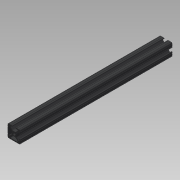
# Autodesk Inventor part: 1002
Saved by Autodesk Inventor 2013 (Build 170138000, 138)
## iProperties
Company: 80/20 Inc.
Created: 2013-09-06
Part Number: 1002
Material: Generic
Document SubType Name: Modeling
Density: 1 g/cm^3
Catalog Web Link: 8020.net
Vendor: 80/20 Inc.
Engineer: Ross Bowman
Author: Ross Bowman
Keywords: T-Slot, Extrusion, 80/20, 8020, Quick Frame, HT
Autodesk Inventor part; units mm, degrees
ref_plane "YZ Plane" through (0, 0, 0) normal (1, 0, 0) x (0, 1, 0)
ref_plane "XZ Plane" through (0, 0, 0) normal (0, 1, 0) x (-1, 0, 0)
ref_plane "XY Plane" through (0, 0, 0) normal (0, 0, 1) x (1, 0, 0)
sketch "Sketch1" plane through (0, 0, 0) normal (0, 0, 1) x (1, 0, 0)
  circle A0 centre (0, 0) radius 2.6035
  arc A1 (-8.737, 7.1292) -> (-10.4902, 6.4021) centre (-9.4628, 6.4021) ccw
  line L0 (-5.4405, 3.8388) -> (-8.737, 7.1292)
  arc A2 (-4.5085, 1.5917) -> (-5.4405, 3.8388) centre (-7.6835, 1.5917) ccw
  line L1 (-4.5085, -1.5917) -> (-4.5085, 1.5917)
  arc A3 (-5.4405, -3.8388) -> (-4.5085, -1.5917) centre (-7.6835, -1.5917) ccw
  line L2 (-8.7534, -7.1457) -> (-5.4405, -3.8388)
  arc A4 (-10.4902, -6.4254) -> (-8.7534, -7.1457) centre (-9.4724, -6.4254) ccw
  line L3 (-10.4902, 6.4021) -> (-10.4902, -6.4254)
  arc A5 (-7.1537, -8.6712) -> (-6.436, -10.4062) centre (-6.436, -9.3902) ccw
  line L4 (-3.9003, -5.4237) -> (-7.1537, -8.6712)
  arc A6 (-1.6573, -4.4958) -> (-3.9003, -5.4237) centre (-1.6573, -7.6708) ccw
  line L5 (1.6573, -4.4958) -> (-1.6573, -4.4958)
  arc A7 (3.9003, -5.4237) -> (1.6573, -4.4958) centre (1.6573, -7.6708) ccw
  line L6 (7.1478, -8.6653) -> (3.9003, -5.4237)
  arc A8 (6.4276, -10.4062) -> (7.1478, -8.6653) centre (6.4276, -9.3868) ccw
  line L7 (-6.436, -10.4062) -> (6.4276, -10.4062)
  arc A9 (6.3331, -12.7) -> (5.3171, -12.7) centre (5.8251, -12.7) ccw
  line L8 (6.3331, -12.7) -> (9.5504, -12.7)
  arc A10 (10.5664, -12.6998) -> (9.5504, -12.7) centre (10.0584, -12.7) ccw
  arc A11 (10.5664, -12.6998) -> (12.6998, -10.5664) centre (10.5918, -10.5918) ccw
  arc A12 (12.7, -9.5504) -> (12.6998, -10.5664) centre (12.7, -10.0584) ccw
  line L9 (12.7, -9.5504) -> (12.7, -6.3331)
  arc A13 (12.7, -5.3171) -> (12.7, -6.3331) centre (12.7, -5.8251) ccw
  line L10 (12.7, -5.3171) -> (12.7, -4.2875)
  arc A14 (12.7, -4.2875) -> (11.651, -3.2385) centre (11.651, -4.2875) ccw
  line L11 (11.651, -3.2385) -> (11.5392, -3.2385)
  arc A15 (11.5392, -3.2385) -> (10.4902, -4.2875) centre (11.5392, -4.2875) ccw
  line L12 (10.4902, -4.2875) -> (10.4902, -6.4021)
  arc A16 (8.737, -7.1292) -> (10.4902, -6.4021) centre (9.4628, -6.4021) ccw
  line L13 (8.737, -7.1292) -> (5.4405, -3.8388)
  arc A17 (4.5085, -1.5917) -> (5.4405, -3.8388) centre (7.6835, -1.5917) ccw
  line L14 (4.5085, -1.5917) -> (4.5085, 1.5917)
  arc A18 (5.4405, 3.8388) -> (4.5085, 1.5917) centre (7.6835, 1.5917) ccw
  line L15 (5.4405, 3.8388) -> (8.737, 7.1292)
  arc A19 (10.4902, 6.4021) -> (8.737, 7.1292) centre (9.4628, 6.4021) ccw
  line L16 (10.4902, 6.4021) -> (10.4902, 4.2875)
  arc A20 (10.4902, 4.2875) -> (11.5392, 3.2385) centre (11.5392, 4.2875) ccw
  line L17 (11.5392, 3.2385) -> (11.651, 3.2385)
  arc A21 (11.651, 3.2385) -> (12.7, 4.2875) centre (11.651, 4.2875) ccw
  line L18 (12.7, 4.2875) -> (12.7, 5.3171)
  arc A22 (12.7, 6.3331) -> (12.7, 5.3171) centre (12.7, 5.8251) ccw
  line L19 (12.7, 6.3331) -> (12.7, 9.5504)
  arc A23 (12.6998, 10.5664) -> (12.7, 9.5504) centre (12.7, 10.0584) ccw
  arc A24 (12.6998, 10.5664) -> (10.5664, 12.6998) centre (10.5918, 10.5918) ccw
  arc A25 (9.5504, 12.7) -> (10.5664, 12.6998) centre (10.0584, 12.7) ccw
  line L20 (9.5504, 12.7) -> (6.3331, 12.7)
  arc A26 (5.3171, 12.7) -> (6.3331, 12.7) centre (5.8251, 12.7) ccw
  line L21 (5.3171, 12.7) -> (4.2875, 12.7)
  arc A27 (4.2875, 12.7) -> (3.2385, 11.651) centre (4.2875, 11.651) ccw
  line L22 (3.2385, 11.651) -> (3.2385, 11.5392)
  arc A28 (3.2385, 11.5392) -> (4.2875, 10.4902) centre (4.2875, 11.5392) ccw
  line L23 (4.2875, 10.4902) -> (6.4768, 10.4902)
  arc A29 (7.2072, 8.7246) -> (6.4768, 10.4902) centre (6.4768, 9.4563) ccw
  line L24 (7.2072, 8.7246) -> (3.9003, 5.4237)
  arc A30 (1.6573, 4.4958) -> (3.9003, 5.4237) centre (1.6573, 7.6708) ccw
  line L25 (1.6573, 4.4958) -> (-1.5537, 4.4958)
  arc A31 (-3.7967, 5.4237) -> (-1.5537, 4.4958) centre (-1.5537, 7.6708) ccw
  line L26 (-3.7967, 5.4237) -> (-7.1342, 8.7551)
  arc A32 (-6.4164, 10.4902) -> (-7.1342, 8.7551) centre (-6.4164, 9.4742) ccw
  line L27 (-6.4164, 10.4902) -> (-4.2875, 10.4902)
  arc A33 (-4.2875, 10.4902) -> (-3.2385, 11.5392) centre (-4.2875, 11.5392) ccw
  line L28 (-3.2385, 11.5392) -> (-3.2385, 11.651)
  arc A34 (-3.2385, 11.651) -> (-4.2875, 12.7) centre (-4.2875, 11.651) ccw
  line L29 (-4.2875, 12.7) -> (-5.3171, 12.7)
  arc A35 (-6.3331, 12.7) -> (-5.3171, 12.7) centre (-5.8251, 12.7) ccw
  line L30 (-6.3331, 12.7) -> (-9.5504, 12.7)
  arc A36 (-10.5664, 12.6998) -> (-9.5504, 12.7) centre (-10.0584, 12.7) ccw
  arc A37 (-10.5664, 12.6998) -> (-12.6998, 10.5664) centre (-10.5918, 10.5918) ccw
  arc A38 (-12.7, 9.5504) -> (-12.6998, 10.5664) centre (-12.7, 10.0584) ccw
  line L31 (-12.7, 9.5504) -> (-12.7, 6.3331)
  arc A39 (-12.7, 5.3171) -> (-12.7, 6.3331) centre (-12.7, 5.8251) ccw
  line L32 (-12.7, 5.3171) -> (-12.7, -5.3171)
  arc A40 (-12.7, -6.3331) -> (-12.7, -5.3171) centre (-12.7, -5.8251) ccw
  line L33 (-12.7, -6.3331) -> (-12.7, -9.5504)
  arc A41 (-12.6998, -10.5664) -> (-12.7, -9.5504) centre (-12.7, -10.0584) ccw
  arc A42 (-12.6998, -10.5664) -> (-10.5664, -12.6998) centre (-10.5918, -10.5918) ccw
  arc A43 (-9.5504, -12.7) -> (-10.5664, -12.6998) centre (-10.0584, -12.7) ccw
  line L34 (-9.5504, -12.7) -> (-6.3331, -12.7)
  arc A44 (-5.3171, -12.7) -> (-6.3331, -12.7) centre (-5.8251, -12.7) ccw
  line L35 (-5.3171, -12.7) -> (5.3171, -12.7)
  constraints: 88 point on circle, 72 end point, 45 centre point
extrude "Extrusion1" add sketch "Sketch1" against normal blind 304.8
body "Solid1"
